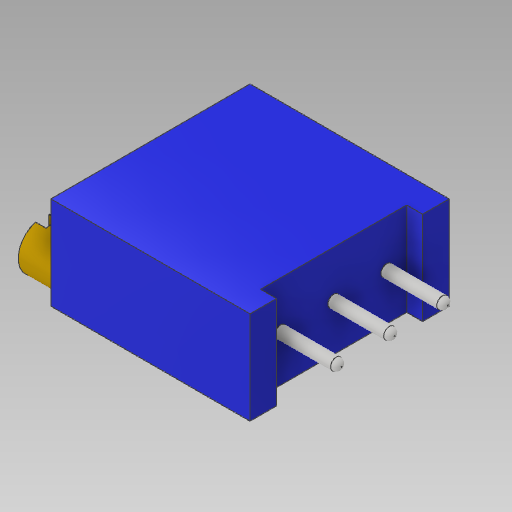
# Autodesk Inventor part: Precision Trim Pot - baoter 3296
Saved by Autodesk Inventor 2020 (Build 240168000, 168)
## iProperties
Created: 2017-07-26
Part Number: Precision Trim Pot - baoter 3296
Material: Generic
Document SubType Name: Modeling
Designer: Alex
Density: 1 g/cm^3
Appearance: Default
Author: Alex
Autodesk Inventor part; units mm, degrees
ref_plane "YZ Plane" through (0, 0, 0) normal (1, 0, 0) x (0, 1, 0)
ref_plane "XZ Plane" through (0, 0, 0) normal (0, 1, 0) x (-1, 0, 0)
ref_plane "XY Plane" through (0, 0, 0) normal (0, 0, 1) x (1, 0, 0)
sketch "Sketch1" plane through (0, 0, 0) normal (0, 1, 0) x (-1, 0, 0)
  line L0 (0, 0) -> (9.525, 0)
  line L1 (9.525, 0) -> (9.525, -9.525)
  line L2 (9.525, -9.525) -> (0, -9.525)
  line L3 (0, -9.525) -> (0, -8.255)
  line L4 (0, -8.255) -> (0.762, -8.255)
  line L5 (0.762, -8.255) -> (0.762, -1.27)
  line L6 (0.762, -1.27) -> (0, -1.27)
  line L7 (0, -1.27) -> (0, 0)
  dimension "d0" = 9.525
  dimension "d1" = 9.525
  dimension "d2" = 6.985
  dimension "d3" = 0.762
  constraints: 16 end point, 7 perpendicular, 1 collinear, 1 horizontal, 1 point on line
  measures "d0" distance of L0.start L0.end
  measures "d1" distance of L0.end L1.end
  measures "d2" distance of L4.end L5.end
  measures "d3" distance of L3.end L4.end
extrude "Extrusion1" add sketch "Sketch1" along normal blind 4.445
sketch "Sketch2" plane through (-0.762, 0, -1.27) normal (1, 0, 0) x (0, 0, -1)
  circle A0 centre (3.4925, 2.2225) radius 0.2794
  circle A1 centre (0.9525, 2.2225) radius 0.2794
  circle A2 centre (6.0325, 2.2225) radius 0.2794
  line L0 (0, 4.445) -> (6.985, 4.445) construction
  line L1 (0, 0) -> (0, 4.445) construction
  point P0 (-1.27, 0)
  point P1 (3.4925, 4.445)
  point P2 (0, 2.2225)
  dimension "d6" = 0.5588
  dimension "d7" = 2.54
  dimension "d8" = 2.54
  constraints: 3 centre point, 3 horizontal alignment, 2 equal radius, 2 midpoint, 1 vertical alignment
  measures "d6" diameter of A0
  measures "d7" distance of A0.centre A1.centre
  measures "d8" distance of A2.centre A0.centre
extrude "Extrusion2" add sketch "Sketch2" along normal blind 2.921
sketch "Sketch3" plane through (-9.525, 0, -9.525) normal (-1, 0, 0) x (0, 0, 1)
  circle A0 centre (8.3566, 1.1684) radius 1.143
  line L0 (9.525, 0) -> (0, 0) projected
  line L1 (9.525, 0) -> (9.525, 4.445) projected
  dimension "d11" = 2.286
  dimension "d12" = 1.1684
  dimension "d13" = 1.1684
  constraints: 1 centre point
  measures "d11" diameter of A0
  measures "d12" distance from line of L0 A0.centre
  measures "d13" distance from line of L1 A0.centre
extrude "Extrusion3" add sketch "Sketch3" along normal blind 1.5875
sketch "Sketch4" plane through (0, 0, 0) normal (0, -1, 0) x (1, 0, 0)
  line L0 (-11.1125, -1.4859) -> (-10.6045, -1.4859)
  line L1 (-10.6045, -1.4859) -> (-10.6045, -0.8509)
  line L2 (-10.6045, -0.8509) -> (-11.1125, -0.8509)
  line L3 (-11.1125, -0.8509) -> (-11.1125, -1.4859)
  line L4 (-11.1125, -0.0254) -> (-11.1125, -2.3114) projected
  point P0 (0, 0)
  point P1 (-11.1125, -1.1684)
  dimension "d16" = 0.508
  dimension "d17" = 0.635
  constraints: 8 end point, 2 midpoint, 2 parallel, 1 horizontal, 1 perpendicular
  measures "d16" distance of L1.end L2.end
  measures "d17" distance of L0.end L1.end
extrude "Extrusion4" cut sketch "Sketch4" against normal through all
fillet "Fillet1" radius 0.254 3 edges at (2.159, 2.2225, -7.0231) (2.159, 2.2225, -4.4831) (2.159, 2.2225, -1.9431)
equation "\"d8\" = d7"
equation "\"d13\" = d12"
body "Solid1"
